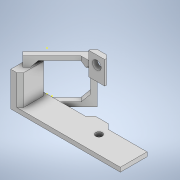
# Autodesk Inventor part: cameraarm
Saved by Autodesk Inventor 2021.2 (Build 252289000, 289)
## iProperties
Created: 2021-03-01
Part Number: cameraarm
Material: Generic
Document SubType Name: Modeling
Designer: zayda
Density: 1 g/cm^3
Appearance: Default
Author: zayda
Autodesk Inventor part; units mm, degrees
ref_plane "YZ Plane" through (0, 0, 0) normal (1, 0, 0) x (0, 1, 0)
ref_plane "XZ Plane" through (0, 0, 0) normal (0, 1, 0) x (-1, 0, 0)
ref_plane "XY Plane" through (0, 0, 0) normal (0, 0, 1) x (1, 0, 0)
sketch "Sketch1" plane through (0, 0, 0) normal (0, 0, 1) x (1, 0, 0)
  line L0 (0, 0) -> (95.25, 0)
  line L1 (95.25, 0) -> (95.25, 4.064)
  line L2 (95.25, 4.064) -> (0, 4.064)
  line L3 (0, 4.064) -> (0, 0)
  line L4 (0, 0) -> (-8.9866, 0)
  line L5 (-8.9866, 0) -> (-8.9866, 18.438)
  line L6 (-8.9866, 18.438) -> (0, 18.438)
  line L7 (0, 18.438) -> (0, 0)
  dimension "d0" = 95.25
  dimension "d1" = 4.064
  constraints: 16 end point, 4 parallel, 2 horizontal, 2 perpendicular
  measures "d0" distance of L2.end L1.end
  measures "d1" distance of L1.end L0.end
extrude "Extrusion1" add sketch "Sketch1" along normal blind 25.4
sketch "Sketch2" plane through (0, 0, 0) normal (0, 0, -1) x (-1, 0, 0)
  line L0 (8.9866, 0) -> (-95.25, 0) projected
  line L1 (-47.4731, 0) -> (-55.0931, 0)
  line L2 (-47.4731, 0) -> (-39.8531, 0)
  line L3 (-55.0931, 0) -> (-55.0931, 45.72)
  line L4 (-55.0931, 45.72) -> (-39.8531, 45.72)
  line L5 (-39.8531, 45.72) -> (-39.8531, 0)
  point P0 (0, 0)
  dimension "d4" = 7.62
  dimension "d5" = 7.62
  dimension "d6" = 45.72
  constraints: 10 end point, 3 point on line, 2 perpendicular, 1 vertical
  measures "d4" distance of L1.start L1.end
  measures "d5" distance of L1.start L2.end
  measures "d6" distance of L1.end L3.end
extrude "Extrusion2" add sketch "Sketch2" along normal blind 4.7625
chamfer "Chamfer1" distance 3.175 angle 45 4 edges at (55.0931, 2.032, 0) (39.8531, 2.032, 0) (39.8531, 22.86, -4.7625) (55.0931, 22.86, -4.7625)
sketch "Sketch3" plane through (39.8531, 45.72, 0) normal (0, 1, 0) x (1, 0, 0)
  line L0 (15.24, 0) -> (0, 0) projected
  line L1 (0, 0) -> (0, 1.5875) projected
  line L2 (15.24, 0) -> (0, 0)
  line L3 (0, 0) -> (0, 1.5875)
  line L4 (0, 1.5875) -> (3.175, 4.7625) projected
  line L5 (0, 1.5875) -> (3.175, 4.7625)
  line L6 (13.6525, 4.7625) -> (12.065, 4.7625) projected
  line L7 (3.175, 4.7625) -> (12.065, 4.7625)
  line L8 (15.24, 0) -> (15.24, 1.5875) projected
  line L9 (12.065, 4.7625) -> (15.24, 1.5875)
  line L10 (15.24, 1.5875) -> (15.24, 0)
  point P0 (-39.8531, 0)
  constraints: 12 end point, 3 perpendicular, 2 collinear, 1 parallel
extrude "Extrusion3" add sketch "Sketch3" along normal blind 14.2875
sketch "Sketch4" plane through (0, 0, -4.7625) normal (0, 0, -1) x (-1, 0, 0)
  circle A0 centre (-47.4731, 51.5851) radius 4.191
  point P0 (0, 0)
  dimension "d14" = 8.382
  constraints: 1 centre point
  measures "d14" diameter of A0
extrude "Extrusion4" cut sketch "Sketch4" against normal blind 14.2875
sketch "Sketch5" plane through (0, 0, -4.7625) normal (0, 0, -1) x (-1, 0, 0)
  point P0 (0, 0)
chamfer "Chamfer2" distance 3.175 angle 45 2 edges at (0, 11.251, 25.4) (0, 11.251, 0)
sketch "Sketch6" plane through (-8.9866, 0, 0) normal (-1, 0, 0) x (0, 0, 1)
  point P0 (0, 0)
sketch "Sketch7" plane through (-8.9866, 18.438, 25.4) normal (0, 1, 0) x (1, 0, 0)
  line L0 (8.9866, 22.225) -> (5.8116, 25.4) projected
  line L1 (8.9866, 22.225) -> (8.9866, 3.175) projected
  line L2 (8.9866, 22.225) -> (8.9866, 3.175)
  line L3 (5.8116, 0) -> (8.9866, 3.175) projected
  line L4 (8.9866, 3.175) -> (5.8116, 0)
  line L5 (5.8116, 0) -> (0, 0) projected
  line L6 (5.8116, 0) -> (0, 0)
  line L7 (0, 25.4) -> (0, 0) projected
  line L8 (0, 0) -> (0, 25.4)
  line L9 (0, 25.4) -> (5.8116, 25.4)
  line L10 (0, 25.4) -> (45.6647, 25.4) projected
  point P0 (8.9866, 25.4)
  constraints: 10 end point, 3 collinear, 1 point on line, 1 vertical
extrude "Extrusion5" add sketch "Sketch7" along normal blind 14.2875
sketch "Sketch8" plane through (-8.9866, 0, 0) normal (-1, 0, 0) x (0, 0, 1)
  point P0 (0, 0)
sketch "Sketch9" plane through (-8.9866, 0, 0) normal (-1, 0, 0) x (0, 0, 1)
  line L0 (22.225, 32.7255) -> (3.175, 32.7255) projected
  line L1 (12.7, 32.7255) -> (12.7, 18.3947)
  line L2 (25.4, 4.064) -> (25.4, 32.7255) projected
  circle A0 centre (12.7, 18.3947) radius 10.3632
  point P0 (0, 0)
  dimension "d22" = 20.7264
  constraints: 2 end point, 1 centre point, 1 coincident, 1 midpoint, 1 parallel
  measures "d22" diameter of A0
extrude "Extrusion6" cut sketch "Sketch9" against normal blind 2.54
sketch "Sketch10" plane through (0, 0, 0) normal (0, 0, 1) x (1, 0, 0)
  line L0 (43.0281, 4.064) -> (43.0281, 60.0075) projected
  line L1 (47.4731, 45.0358) -> (52.8994, 45.0358) construction
  line L2 (43.0281, 41.9234) -> (43.0281, 4.064)
  line L3 (55.0931, 4.064) -> (39.8531, 4.064) projected
  line L4 (51.9181, 4.064) -> (51.9181, 60.0075) projected
  line L5 (51.9181, 4.064) -> (43.0281, 4.064)
  line L6 (51.9181, 41.9234) -> (43.0281, 41.9234)
  point P0 (0, 0)
  constraints: 8 end point, 4 point on line, 1 collinear, 1 horizontal, 1 perpendicular, 1 vertical
extrude "Extrusion7" [suppressed]
sketch "Sketch11" plane through (95.25, 4.064, 25.4) normal (0, 1, 0) x (1, 0, 0)
  point P0 (-95.25, 25.4)
sketch "Sketch12" plane through (39.8531, 4.064, -1.5875) normal (-0.7071068, 0, -0.7071068) x (-0.7071068, 0, 0.7071068)
  line L0 (-1.1225, 37.8594) -> (-4.4901, 37.8594) projected
  line L1 (0, 0) -> (0, 55.9435) projected
  line L2 (-4.4901, 37.8594) -> (0, 37.8594)
  line L3 (0, 37.8594) -> (0, 34.028)
  line L4 (0, 34.028) -> (-4.4901, 34.028)
  line L5 (-4.4901, 34.028) -> (-4.4901, 37.8594)
  point P0 (29.3029, -4.064)
  point P1 (0, 37.8594)
  constraints: 8 end point, 2 parallel, 1 horizontal, 1 perpendicular, 1 point on line
extrude "Extrusion8" add sketch "Sketch12" along normal blind 23.1775
sketch "Sketch13" plane through (39.8531, 38.092, -1.5875) normal (-0.7071068, 0, 0.7071068) x (0.7071068, 0, 0.7071068)
  line L0 (-23.1775, 0) -> (-23.1775, 3.8313) projected
  line L1 (0, 0) -> (-23.1775, 0) projected
  line L2 (-23.1775, 3.8313) -> (-17.8376, 3.8313)
  line L3 (-17.8376, 3.8313) -> (-17.8376, 0)
  line L4 (-17.8376, 0) -> (-23.1775, 0)
  line L5 (-23.1775, 0) -> (-23.1775, 3.8313)
  point P0 (-27.0579, -38.092)
  constraints: 8 end point, 2 parallel, 1 horizontal, 1 perpendicular, 1 point on line
extrude "Extrusion9" add sketch "Sketch13" along normal blind 45.4025
sketch "Sketch14" plane through (43.0281, 38.092, -4.7625) normal (0, -1, 0) x (0.7071068, 0, 0.7071068)
  line L0 (-23.1775, 49.8926) -> (-17.8376, 49.8926) projected
  line L1 (-17.8376, 4.4901) -> (-17.8376, 49.8926) projected
  line L2 (-23.1775, 49.8926) -> (-17.8376, 49.8926)
  line L3 (-17.8376, 49.8926) -> (-17.8376, 44.3958)
  line L4 (-17.8376, 44.3958) -> (-23.1775, 44.3958)
  line L5 (-23.1775, 44.3958) -> (-23.1775, 49.8926)
  point P0 (-27.0579, 33.7931)
  constraints: 8 end point, 2 parallel, 1 horizontal, 1 perpendicular, 1 point on line
extrude "Extrusion10" add sketch "Sketch14" along normal blind 5.715
sketch "Sketch15" plane through (43.0281, 4.064, 0) normal (1, 0, 0) x (0, 0, -1)
  line L0 (4.7625, 0) -> (4.7625, 34.028) projected
  line L1 (0, 0) -> (0, 37.8594) projected
  line L2 (4.7625, 34.028) -> (0, 34.028)
  line L3 (0, 34.028) -> (0, 37.8594)
  line L4 (0, 37.8594) -> (4.7625, 37.8594)
  line L5 (4.7625, 37.8594) -> (4.7625, 34.028)
  point P0 (0, -4.064)
  constraints: 8 end point, 2 parallel, 1 horizontal, 1 perpendicular
extrude "Extrusion11" [suppressed]
sketch "Sketch16" plane through (43.0281, 41.9234, 0) normal (0, 1, 0) x (1, 0, 0)
  point P0 (-43.0281, 0)
sketch "Sketch17" plane through (0, 0, -4.7625) normal (0, 0, -1) x (-1, 0, 0)
  line L0 (-39.8531, 4.064) -> (-39.8531, 38.092) projected
  line L1 (-55.0931, 60.0075) -> (-55.0931, 4.064) projected
  line L2 (-39.8531, 38.092) -> (-55.0931, 38.092)
  line L3 (-55.0931, 38.092) -> (-55.0931, 4.064)
  line L4 (-55.0931, 4.064) -> (-39.8531, 4.064)
  line L5 (-39.8531, 4.064) -> (-39.8531, 38.092)
  point P0 (0, 0)
  constraints: 8 end point, 2 parallel, 1 horizontal, 1 perpendicular
extrude "Extrusion12" cut sketch "Sketch17" against normal blind 536267.66
sketch "Sketch18" plane through (39.8531, 38.092, 0) normal (0, -1, 0) x (1, 0, 0)
  line L0 (-12.6131, -14.2006) -> (-40.8307, 14.017) projected
  line L1 (-12.6131, -14.2006) -> (-9.4381, -17.3756)
  line L2 (3.175, -4.7625) -> (-13.214, -21.1515) projected
  line L3 (-12.6131, -14.2006) -> (-16.389, -17.9765)
  line L4 (-13.214, -21.1515) -> (-44.6066, 10.2411) projected
  line L5 (-13.214, -21.1515) -> (-9.4381, -17.3756)
  line L6 (-16.389, -17.9765) -> (-13.214, -21.1515)
  point P0 (-39.8531, 0)
  constraints: 8 end point, 3 point on line, 2 perpendicular, 1 parallel
extrude "Extrusion13" add sketch "Sketch18" along normal blind 38.1
sketch "Sketch19" plane through (23.4641, -0.008, -17.9765) normal (-0.7071068, 0, 0.7071068) x (0.7071068, 0, 0.7071068)
  line L0 (5.3399, 0) -> (0, 0) projected
  line L1 (0, 0) -> (4.064, 0)
  line L2 (4.064, 0) -> (4.064, 4.064)
  line L3 (4.064, 4.064) -> (0, 4.064)
  line L4 (0, 4.064) -> (0, 0)
  line L5 (4.064, 4.064) -> (5.3399, 4.064)
  line L6 (5.3399, 38.1) -> (5.3399, 0) projected
  line L7 (5.3399, 0) -> (4.064, 0)
  point P0 (-3.8804, 0.008)
  dimension "d41" = 4.064
  constraints: 12 end point, 2 horizontal, 2 parallel, 1 collinear, 1 perpendicular, 1 point on line
  measures "d41" distance of L2.end L1.end
extrude "Extrusion14" add sketch "Sketch19" along normal blind 25.654
chamfer "Chamfer3" distance 6.35 angle 45 4 edges at (27.24, 40.0077, -14.2006) (28.8275, 38.092, -15.7881) (25.3521, 38.092, -16.0885) (25.3521, 4.056, -16.0885)
chamfer "Chamfer4" distance 4.7625 angle 45 1 edges at (-2.8655, 38.092, 12.1291)
sketch "Sketch20" plane through (95.25, 4.064, 25.4) normal (0, 1, 0) x (1, 0, 0)
  line L0 (-95.25, 22.225) -> (-95.25, 3.175) projected
  line L1 (0, 25.4) -> (0, 0) projected
  line L2 (-82.2106, 25.4) -> (-58.5719, 25.4) projected
  line L3 (0, 25.4) -> (-36.9819, 25.4) projected
  line L4 (-60.4109, 58.42) -> (-60.4109, 25.4)
  circle A0 centre (-37.1699, 16.8767) radius 3.175
  point P0 (-95.25, 25.4)
  dimension "d53" = 6.35
  constraints: 2 end point, 1 centre point
  measures "d53" diameter of A0
extrude "Extrusion15" cut sketch "Sketch20" against normal blind 25.4
body "Solid1"
